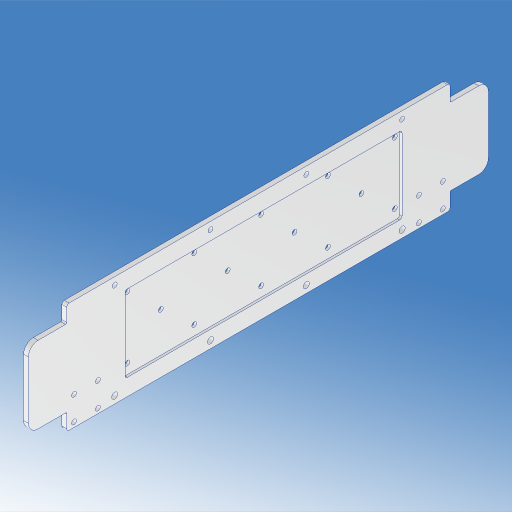
# Autodesk Inventor part: ChassisInterface
Saved by Autodesk Inventor 2024 (Build 280153000, 153)
## iProperties
Created: 2022-11-13
Part Number: ChassisInterface
Material: Aluminum 6061
Document SubType Name: Modeling
Designer: kumpu
Density: 2.7 g/cm^3
Appearance: Aluminum - Flat
Mass: 777.044 g
Surface Area: 1099.09 cm^2
Volume: 287.794 cm^3
Author: kumpu
Autodesk Inventor part; units mm, degrees
ref_plane "YZ Plane" through (0, 0, 0) normal (1, 0, 0) x (0, 1, 0)
ref_plane "XZ Plane" through (0, 0, 0) normal (0, 1, 0) x (-1, 0, 0)
ref_plane "XY Plane" through (0, 0, 0) normal (0, 0, 1) x (1, 0, 0)
sketch "Sketch1" plane through (0, 0, 0) normal (1, 0, 0) x (0, 1, 0)
  line L0 (76.2, 254) -> (-76.2, 254)
  line L1 (-76.2, 254) -> (-76.2, -254)
  line L2 (-76.2, -254) -> (76.2, -254)
  line L3 (76.2, -254) -> (76.2, 254)
  line L4 (76.2, 254) -> (-76.2, -254) construction
  line L5 (-76.2, 254) -> (76.2, -254) construction
  line L6 (50.8, 304.8) -> (-50.8, 304.8)
  line L7 (-50.8, 304.8) -> (-50.8, 254)
  line L8 (-50.8, 254) -> (50.8, 254)
  line L9 (50.8, 254) -> (50.8, 304.8)
  line L10 (50.8, 304.8) -> (-50.8, 254) construction
  line L11 (-50.8, 304.8) -> (50.8, 254) construction
  line L12 (50.8, -254) -> (-50.8, -254)
  line L13 (-50.8, -254) -> (-50.8, -304.8)
  line L14 (-50.8, -304.8) -> (50.8, -304.8)
  line L15 (50.8, -304.8) -> (50.8, -254)
  line L16 (50.8, -254) -> (-50.8, -304.8) construction
  line L17 (-50.8, -254) -> (50.8, -304.8) construction
  line L18 (0, 279.4) -> (0, -279.4) construction
  point P0 (0, 0)
  point P1 (-50.8, -254)
  point P2 (50.8, 254)
  dimension "d0" = 152.4
  dimension "d1" = 508
  dimension "d9" = 50.8
  dimension "d10" = 101.6
  constraints: 38 end point, 7 midpoint, 6 parallel, 3 horizontal, 3 perpendicular, 2 equal length, 1 point on line, 1 vertical
  measures "d0" distance of L2.end L1.end
  measures "d1" distance of L1.end L0.end
  measures "d9" distance of L14.end L12.start
  measures "d10" distance of L13.end L14.end
extrude "Extrusion1" add sketch "Sketch1" along normal mid plane 6.35
sketch "Sketch3" plane through (3.175, 0, 0) normal (1, 0, 0) x (0, 0, -1)
  line L0 (-241.3, 44.45) -> (-201.6125, 44.45)
  line L1 (-201.6125, 44.45) -> (-201.6125, -44.45)
  line L2 (-201.6125, -44.45) -> (-241.3, -44.45)
  line L3 (-241.3, -44.45) -> (-241.3, 44.45)
  line L4 (-179.3875, 44.45) -> (-125.857, 44.45)
  line L5 (-125.857, 44.45) -> (-125.857, -44.45)
  line L6 (-125.857, -44.45) -> (-179.3875, -44.45)
  line L7 (-179.3875, -44.45) -> (-179.3875, 44.45)
  line L8 (-103.632, 44.45) -> (50.8, 44.45)
  line L9 (50.8, 44.45) -> (50.8, -44.45)
  line L10 (50.8, -44.45) -> (-103.632, -44.45)
  line L11 (-103.632, -44.45) -> (-103.632, 44.45)
  line L12 (74.6125, 44.45) -> (179.3875, 44.45)
  line L13 (179.3875, 44.45) -> (179.3875, -44.45)
  line L14 (179.3875, -44.45) -> (74.6125, -44.45)
  line L15 (74.6125, -44.45) -> (74.6125, 44.45)
  line L16 (201.6125, -44.45) -> (241.3, -44.45)
  line L17 (241.3, -44.45) -> (241.3, 44.45)
  line L18 (241.3, 44.45) -> (201.6125, 44.45)
  line L19 (201.6125, 44.45) -> (201.6125, -44.45)
  line L20 (-201.6125, 0) -> (-179.3875, 0) construction
  line L21 (-125.857, 0) -> (-103.632, 0) construction
  line L22 (179.3875, 0) -> (201.6125, 0) construction
  line L23 (-254, -50.8) -> (-254, -76.2) construction
  circle A0 centre (-190.5, 63.5) radius 3.175
  line L24 (-190.5, 63.5) -> (-190.5, 0) construction
  line L25 (-190.5, 0) -> (-190.5, -63.5) construction
  circle A1 centre (-190.5, -63.5) radius 3.9751
  circle A2 centre (-63.5, 63.5) radius 3.175
  circle A3 centre (-63.5, -63.5) radius 3.9751
  circle A4 centre (63.5, 63.5) radius 3.175
  circle A5 centre (63.5, -63.5) radius 3.9751
  circle A6 centre (190.5, 63.5) radius 3.175
  circle A7 centre (190.5, -63.5) radius 3.9751
  line L26 (-125.857, 44.45) -> (-103.632, 44.45)
  line L27 (-103.632, 44.45) -> (-103.632, -44.45)
  line L28 (-103.632, -44.45) -> (-125.857, -44.45)
  line L29 (-125.857, -44.45) -> (-125.857, 44.45)
  line L30 (254, -76.2) -> (254, -50.8) projected
  line L31 (-254, -76.2) -> (254, -76.2) projected
  point P0 (0, 0)
  point P1 (0, 0)
  point P2 (-114.7445, 0)
  dimension "d12" = 22.225
  dimension "d13" = 12.7
  dimension "d14" = 88.9
  dimension "d16" = 6.35
  dimension "d17" = 7.9502
  dimension "d20" = 127
  dimension "d29" = 12.7
  dimension "d30" = 63.5
  dimension "d31" = 12.7
  dimension "d32" = 11.1125
  dimension "d33" = 31.75
  dimension "d34" = 127
  dimension "d35" = 63.5
  dimension "d39" = 154.432
  constraints: 58 end point, 12 parallel, 8 centre point, 8 midpoint, 7 collinear, 7 horizontal, 7 perpendicular, 4 point on line, 2 coincident, 1 vertical, 12 other
  measures "d12" distance of L20.start L20.end
  measures "d13" distance between parallel lines of L23 L3
  measures "d14" distance of L2.end L0.start
  measures "d16" diameter of A0
  measures "d17" diameter of A1
  measures "d20" distance of L24.start A2.centre
  measures "d29" distance from line of L9 A4.centre
  measures "d30" distance between parallel lines of L23 L25
  measures "d31" distance between parallel lines of L30 L17
  measures "d32" distance from line of A4.centre L15
  measures "d33" distance between parallel lines of L31 L2
  measures "d34" distance of L25.end L24.start
  measures "d35" distance from line of L20 L24.start
  measures "d39" distance between parallel lines of L9 L27
extrude "Extrusion3" [suppressed]
fillet "Fillet1" radius 12.7 4 edges at (0, 50.8, 304.8) (0, -50.8, 304.8) (0, 50.8, -304.8) (0, -50.8, -304.8)
fillet "Fillet1" radius 1.5875 8 edges at (0, 50.8, 254) (0, -50.8, 254) (0, -76.2, 254) (0, 76.2, 254) (0, 76.2, -254) (0, 50.8, -254) (0, -50.8, -254) (0, -76.2, -254)
sketch "Sketch4" plane through (-3.175, 0, 0) normal (-1, 0, 0) x (0, 0, 1)
  line L0 (-182.626, 63.5635) -> (-141.351, 63.5635) construction
  line L1 (-254, 74.6125) -> (-254, 52.3875) construction
  line L2 (252.4125, 76.2) -> (-252.4125, 76.2) construction
  point P0 (0, 0)
  dimension "d36" = 71.374
  dimension "d37" = 12.6365
  dimension "d38" = 41.275
  constraints: 2 end point, 1 horizontal
  measures "d36" distance from line of L1 L0.start
  measures "d37" distance between parallel lines of L2 L0
  measures "d38" distance of L0.start L0.end
extrude "Extrusion4" cut sketch "Sketch3" against normal through all contours A0 | A1 | A2 | A3 | A4 | A5 | A6 | A7
sketch "Sketch6" plane through (3.175, 0, 0) normal (1, 0, 0) x (0, 0, -1)
  circle A0 centre (63.5, 63.5) radius 3.175 projected
  circle A1 centre (-63.5, -63.5) radius 3.9751 projected
  circle A2 centre (63.5, -63.5) radius 3.9751 projected
  circle A3 centre (-63.5, 63.5) radius 3.175 projected
  circle A4 centre (190.5, 63.5) radius 3.175 projected
  circle A5 centre (-190.5, -63.5) radius 3.9751 projected
  circle A6 centre (190.5, -63.5) radius 3.9751 projected
  circle A7 centre (-190.5, 63.5) radius 3.175 projected
  arc A8 (252.4125, -76.2) -> (254, -74.6125) centre (252.4125, -74.6125) ccw projected
  line L0 (254, -74.6125) -> (254, -52.3875) projected
  arc A9 (255.5875, -50.8) -> (254, -52.3875) centre (255.5875, -52.3875) ccw projected
  line L1 (255.5875, -50.8) -> (292.1, -50.8) projected
  arc A10 (292.1, -50.8) -> (304.8, -38.1) centre (292.1, -38.1) ccw projected
  line L2 (304.8, -38.1) -> (304.8, 38.1) projected
  arc A11 (304.8, 38.1) -> (292.1, 50.8) centre (292.1, 38.1) ccw projected
  line L3 (292.1, 50.8) -> (255.5875, 50.8) projected
  arc A12 (254, 52.3875) -> (255.5875, 50.8) centre (255.5875, 52.3875) ccw projected
  line L4 (254, 52.3875) -> (254, 74.6125) projected
  arc A13 (254, 74.6125) -> (252.4125, 76.2) centre (252.4125, 74.6125) ccw projected
  line L5 (252.4125, 76.2) -> (-252.4125, 76.2) projected
  arc A14 (-252.4125, 76.2) -> (-254, 74.6125) centre (-252.4125, 74.6125) ccw projected
  line L6 (-254, 74.6125) -> (-254, 52.3875) projected
  arc A15 (-255.5875, 50.8) -> (-254, 52.3875) centre (-255.5875, 52.3875) ccw projected
  line L7 (-255.5875, 50.8) -> (-292.1, 50.8) projected
  arc A16 (-292.1, 50.8) -> (-304.8, 38.1) centre (-292.1, 38.1) ccw projected
  line L8 (-304.8, 38.1) -> (-304.8, -38.1) projected
  arc A17 (-304.8, -38.1) -> (-292.1, -50.8) centre (-292.1, -38.1) ccw projected
  line L9 (-292.1, -50.8) -> (-255.5875, -50.8) projected
  arc A18 (-254, -52.3875) -> (-255.5875, -50.8) centre (-255.5875, -52.3875) ccw projected
  line L10 (-254, -52.3875) -> (-254, -74.6125) projected
  arc A19 (-254, -74.6125) -> (-252.4125, -76.2) centre (-252.4125, -74.6125) ccw projected
  line L11 (-252.4125, -76.2) -> (252.4125, -76.2) projected
  line L12 (-292.1, 47.625) -> (-255.5875, 47.625)
  arc A20 (-255.5875, 47.625) -> (-250.825, 52.3875) centre (-255.5875, 52.3875) ccw
  line L13 (-250.825, 52.3875) -> (-250.825, 73.025)
  line L14 (-250.825, 73.025) -> (250.825, 73.025)
  line L15 (250.825, 73.025) -> (250.825, 52.3875)
  arc A21 (250.825, 52.3875) -> (255.5875, 47.625) centre (255.5875, 52.3875) ccw
  line L16 (255.5875, 47.625) -> (292.1, 47.625)
  arc A22 (301.625, 38.1) -> (292.1, 47.625) centre (292.1, 38.1) ccw
  line L17 (301.625, 38.1) -> (301.625, -38.1)
  arc A23 (292.1, -47.625) -> (301.625, -38.1) centre (292.1, -38.1) ccw
  line L18 (292.1, -47.625) -> (255.5875, -47.625)
  arc A24 (255.5875, -47.625) -> (250.825, -52.3875) centre (255.5875, -52.3875) ccw
  line L19 (250.825, -52.3875) -> (250.825, -73.025)
  line L20 (250.825, -73.025) -> (-250.825, -73.025)
  line L21 (-250.825, -73.025) -> (-250.825, -52.3875)
  arc A25 (-250.825, -52.3875) -> (-255.5875, -47.625) centre (-255.5875, -52.3875) ccw
  line L22 (-255.5875, -47.625) -> (-292.1, -47.625)
  arc A26 (-301.625, -38.1) -> (-292.1, -47.625) centre (-292.1, -38.1) ccw
  line L23 (-301.625, -38.1) -> (-301.625, 38.1)
  arc A27 (-292.1, 47.625) -> (-301.625, 38.1) centre (-292.1, 38.1) ccw
  line L24 (-295.0658, 0) -> (-301.625, 0) construction
  line L25 (-176.784, 50.8) -> (190.3494, 50.8)
  line L26 (190.3494, 50.8) -> (190.3494, -50.8)
  line L27 (190.3494, -50.8) -> (-176.784, -50.8)
  line L28 (-176.784, -50.8) -> (-176.784, 50.8)
  line L29 (-254, -50.8) -> (254, -50.8) construction
  line L30 (254, -50.8) -> (254, -76.2) construction
  line L31 (254, -76.2) -> (-254, -76.2) construction
  line L32 (-254, -76.2) -> (-254, -50.8) construction
  line L33 (-254, 76.2) -> (254, 76.2) construction
  line L34 (254, 76.2) -> (254, 50.8) construction
  line L35 (254, 50.8) -> (-254, 50.8) construction
  line L36 (-254, 50.8) -> (-254, 76.2) construction
  circle A28 centre (-170.434, 44.45) radius 3.302
  circle A29 centre (183.9994, 44.45) radius 3.175
  circle A30 centre (-81.8256, 44.45) radius 3.175
  circle A31 centre (6.7827, 44.45) radius 3.175
  circle A32 centre (95.3911, 44.45) radius 3.175
  line L37 (-330.2, 73.025) -> (-330.2, -50.8) construction
  circle A33 centre (-37.5215, 1.7998) radius 3.175
  circle A34 centre (51.0869, 1.7998) radius 3.175
  line L38 (639.9011, -38.0592) -> (645.7898, -37.8143) construction
  circle A35 centre (228.6, -50.8) radius 12.7 construction
  circle A36 centre (-228.6, -50.8) radius 12.7 construction
  circle A37 centre (-228.6, -50.8) radius 15.875 construction
  line L39 (-244.475, -34.925) -> (-212.725, -34.925) construction
  line L40 (-212.725, -34.925) -> (-212.725, -66.675) construction
  line L41 (-212.725, -66.675) -> (-244.475, -66.675) construction
  line L42 (-244.475, -66.675) -> (-244.475, -34.925) construction
  circle A38 centre (228.6, -50.8) radius 15.875 construction
  line L43 (212.725, -34.925) -> (244.475, -34.925) construction
  line L44 (244.475, -34.925) -> (244.475, -66.675) construction
  line L45 (244.475, -66.675) -> (212.725, -66.675) construction
  line L46 (212.725, -66.675) -> (212.725, -34.925) construction
  circle A39 centre (-244.475, -34.925) radius 3.175
  circle A40 centre (-244.475, -66.675) radius 3.175
  circle A41 centre (-212.725, -66.675) radius 3.175
  circle A42 centre (-212.725, -34.925) radius 3.175
  circle A43 centre (212.725, -34.925) radius 3.175
  circle A44 centre (244.475, -34.925) radius 3.175
  circle A45 centre (212.725, -66.675) radius 3.175
  circle A46 centre (244.475, -66.675) radius 3.175
  line L47 (643.6065, -35.788) -> (639.9011, -38.0592) construction
  line L48 (6.7827, 50.8) -> (6.7827, -50.8) construction
  circle A47 centre (-126.1298, 1.7998) radius 3.175
  circle A48 centre (139.6953, 1.7998) radius 3.175
  circle A49 centre (-37.5215, 1.7998) radius 3.175
  circle A50 centre (51.0869, 1.7998) radius 3.175
  circle A51 centre (-126.1298, 1.7998) radius 3.175
  circle A52 centre (139.6953, 1.7998) radius 3.175
  circle A53 centre (-170.434, -37.6754) radius 3.175
  circle A54 centre (-81.8256, -37.6754) radius 3.175
  circle A55 centre (6.7827, -37.6754) radius 3.175
  circle A56 centre (95.3911, -37.6754) radius 3.175
  circle A57 centre (183.9994, -37.6754) radius 3.175
  dimension "d42" = 3.175
  dimension "d57" = 101.6
  dimension "d58" = 25.4
  dimension "d59" = 25.4
  dimension "d60" = 367.1334
  dimension "d61" = 6.35
  dimension "d62" = 6.35
  dimension "d63" = 6.35
  dimension "d64" = 6.35
  dimension "d65" = 6.604
  dimension "d66" = 6.35
  dimension "d69" = 6.35
  dimension "d70" = 6.35
  dimension "d71" = 6.35
  dimension "d73" = 25.4
  dimension "d82" = 6.35
  dimension "d84" = 6.35
  dimension "d119" = 25.4
  dimension "d120" = 25.4
  dimension "d121" = 76.2
  dimension "d124" = 25.4
  dimension "d125" = 76.2
  dimension "d126" = 25.4
  dimension "d127" = 3.175
  dimension "d128" = 3.175
  dimension "d129" = 6.35
  dimension "d130" = 6.35
  dimension "d131" = 6.35
  dimension "d132" = 6.35
  dimension "d133" = 6.35
  dimension "d134" = 6.35
  dimension "d135" = 6.35
  dimension "d136" = 6.35
  dimension "d139" = 177.2167
  dimension "d140" = 88.6084
  dimension "d141" = 88.6084
  dimension "d142" = 6.35
  dimension "d143" = 6.35
  dimension "d144" = 44.3042
  dimension "d145" = 44.3042
  dimension "d146" = 44.3042
  dimension "d147" = 44.3042
  dimension "d148" = 38.2506
  dimension "d149" = 6.35
  dimension "d151" = 6.35
  dimension "d152" = 6.35
  dimension "d153" = 6.35
  dimension "d154" = 6.35
  dimension "d155" = 42.6502
  dimension "d156" = 82.1254
  constraints: 74 end point, 38 centre point, 16 point on circle, 10 horizontal alignment, 10 parallel, 8 coincident, 8 tangent, 7 collinear, 6 horizontal, 5 perpendicular, 4 vertical alignment, 3 midpoint, 2 point on line, 1 vertical, 19 other
  measures "d42" distance between parallel lines of L7 L12
  measures "d57" distance of L25.end L26.end
  measures "d58" distance of L29.end L30.end
  measures "d59" distance of L35.end L33.start
  measures "d60" distance between parallel lines of L26 L28
  measures "d61" distance from line of L28 A28.centre
  measures "d62" distance from line of L35 A28.centre
  measures "d63" distance from line of L25 A29.centre
  measures "d64" distance from line of L26 A29.centre
  measures "d65" diameter of A28
  measures "d66" diameter of A29
  measures "d69" diameter of A30
  measures "d70" diameter of A31
  measures "d71" diameter of A32
  measures "d73" distance between parallel lines of L8 L37
  measures "d82" diameter of A33
  measures "d84" diameter of A34
  measures "d119" diameter of A35
  measures "d120" distance from line of L11 A35.centre
  measures "d121" distance from line of A35.centre L2
  measures "d124" diameter of A36
  measures "d125" distance from line of A36.centre L8
  measures "d126" distance from line of L11 A36.centre
  measures "d127" radial gap between concentric circles of A36 A37
  measures "d128" radial gap between concentric circles of A35 A38
  measures "d129" diameter of A39
  measures "d130" diameter of A40
  measures "d131" diameter of A41
  measures "d132" diameter of A42
  measures "d133" diameter of A43
  measures "d134" diameter of A44
  measures "d135" diameter of A45
  measures "d136" diameter of A46
  measures "d139" distance of A31.centre A28.centre
  measures "d140" distance of A30.centre A28.centre
  measures "d141" distance of A32.centre A31.centre
  measures "d142" diameter of A47
  measures "d143" diameter of A48
  measures "d144" horizontal distance of A47.centre A28.centre
  measures "d145" horizontal distance of A33.centre A30.centre
  measures "d146" horizontal distance of A34.centre A31.centre
  measures "d147" horizontal distance of A48.centre A32.centre
  measures "d148" distance from line of A35.centre L26
  measures "d149" diameter of A53
  measures "d151" diameter of A54
  measures "d152" diameter of A55
  measures "d153" diameter of A56
  measures "d154" diameter of A57
  measures "d155" vertical distance of A47.centre A28.centre
  measures "d156" distance of A53.centre A28.centre
extrude "Extrusion5" cut sketch "Sketch6" against normal blind 25.4 contours A28 | A29 | A30 | A31 | A32 | A33 | A34 | A47 | A48 | A53 | A54 | A55 | A56 | A57
extrude "Extrusion6" cut sketch "Sketch6" against normal blind 3.175 contours L25 L26 L27 L28 | A28 | A29 | A30 | A31 | A32 | A33 | A34 | A47 | A48 | A53 | A54 | A55 | A56 | A57
sketch "Sketch7" plane through (3.175, 0, 0) normal (1, 0, 0) x (0, 0, -1)
  line L0 (190.3494, 50.8) -> (190.3494, -50.8) projected
  line L1 (190.3494, -50.8) -> (-176.784, -50.8) projected
  line L2 (-176.784, -50.8) -> (-176.784, 50.8) projected
  line L3 (-176.784, 50.8) -> (190.3494, 50.8) projected
  circle A0 centre (63.5, 63.5) radius 3.175 projected
  circle A1 centre (-63.5, -63.5) radius 3.9751 projected
  circle A2 centre (63.5, -63.5) radius 3.9751 projected
  circle A3 centre (-63.5, 63.5) radius 3.175 projected
  circle A4 centre (190.5, 63.5) radius 3.175 projected
  circle A5 centre (-190.5, -63.5) radius 3.9751 projected
  circle A6 centre (190.5, -63.5) radius 3.9751 projected
  circle A7 centre (-190.5, 63.5) radius 3.175 projected
  arc A8 (252.4125, -76.2) -> (254, -74.6125) centre (252.4125, -74.6125) ccw projected
  line L4 (254, -74.6125) -> (254, -52.3875) projected
  arc A9 (255.5875, -50.8) -> (254, -52.3875) centre (255.5875, -52.3875) ccw projected
  line L5 (255.5875, -50.8) -> (292.1, -50.8) projected
  arc A10 (292.1, -50.8) -> (304.8, -38.1) centre (292.1, -38.1) ccw projected
  line L6 (304.8, -38.1) -> (304.8, 38.1) projected
  arc A11 (304.8, 38.1) -> (292.1, 50.8) centre (292.1, 38.1) ccw projected
  line L7 (292.1, 50.8) -> (255.5875, 50.8) projected
  arc A12 (254, 52.3875) -> (255.5875, 50.8) centre (255.5875, 52.3875) ccw projected
  line L8 (254, 52.3875) -> (254, 74.6125) projected
  arc A13 (254, 74.6125) -> (252.4125, 76.2) centre (252.4125, 74.6125) ccw projected
  line L9 (252.4125, 76.2) -> (-252.4125, 76.2) projected
  arc A14 (-252.4125, 76.2) -> (-254, 74.6125) centre (-252.4125, 74.6125) ccw projected
  line L10 (-254, 74.6125) -> (-254, 52.3875) projected
  arc A15 (-255.5875, 50.8) -> (-254, 52.3875) centre (-255.5875, 52.3875) ccw projected
  line L11 (-255.5875, 50.8) -> (-292.1, 50.8) projected
  arc A16 (-292.1, 50.8) -> (-304.8, 38.1) centre (-292.1, 38.1) ccw projected
  line L12 (-304.8, 38.1) -> (-304.8, -38.1) projected
  arc A17 (-304.8, -38.1) -> (-292.1, -50.8) centre (-292.1, -38.1) ccw projected
  line L13 (-292.1, -50.8) -> (-255.5875, -50.8) projected
  arc A18 (-254, -52.3875) -> (-255.5875, -50.8) centre (-255.5875, -52.3875) ccw projected
  line L14 (-254, -52.3875) -> (-254, -74.6125) projected
  arc A19 (-254, -74.6125) -> (-252.4125, -76.2) centre (-252.4125, -74.6125) ccw projected
  line L15 (-252.4125, -76.2) -> (252.4125, -76.2) projected
  line L16 (-250.825, 52.3875) -> (-250.825, 73.025)
  line L17 (-250.825, 73.025) -> (250.825, 73.025)
  line L18 (250.825, 73.025) -> (250.825, 52.3875)
  arc A20 (250.825, 52.3875) -> (255.5875, 47.625) centre (255.5875, 52.3875) ccw
  line L19 (255.5875, 47.625) -> (292.1, 47.625)
  arc A21 (301.625, 38.1) -> (292.1, 47.625) centre (292.1, 38.1) ccw
  line L20 (301.625, 38.1) -> (301.625, -38.1)
  arc A22 (292.1, -47.625) -> (301.625, -38.1) centre (292.1, -38.1) ccw
  line L21 (292.1, -47.625) -> (255.5875, -47.625)
  arc A23 (255.5875, -47.625) -> (250.825, -52.3875) centre (255.5875, -52.3875) ccw
  line L22 (250.825, -52.3875) -> (250.825, -73.025)
  line L23 (250.825, -73.025) -> (-250.825, -73.025)
  line L24 (-250.825, -73.025) -> (-250.825, -52.3875)
  arc A24 (-250.825, -52.3875) -> (-255.5875, -47.625) centre (-255.5875, -52.3875) ccw
  line L25 (-255.5875, -47.625) -> (-292.1, -47.625)
  arc A25 (-301.625, -38.1) -> (-292.1, -47.625) centre (-292.1, -38.1) ccw
  line L26 (-301.625, -38.1) -> (-301.625, 38.1)
  arc A26 (-292.1, 47.625) -> (-301.625, 38.1) centre (-292.1, 38.1) ccw
  line L27 (-292.1, 47.625) -> (-255.5875, 47.625)
  arc A27 (-255.5875, 47.625) -> (-250.825, 52.3875) centre (-255.5875, 52.3875) ccw
  line L28 (196.6994, 57.15) -> (196.6994, -57.15)
  line L29 (196.6994, -57.15) -> (-183.134, -57.15)
  line L30 (-183.134, -57.15) -> (-183.134, 57.15)
  line L31 (-183.134, 57.15) -> (196.6994, 57.15)
  circle A28 centre (-190.5, 63.5) radius 6.35
  circle A29 centre (-63.5, 63.5) radius 6.35
  circle A30 centre (63.5, 63.5) radius 6.35
  circle A31 centre (190.5, 63.5) radius 6.35
  circle A32 centre (-190.5, -63.5) radius 6.35
  circle A33 centre (-63.5, -63.5) radius 6.35
  circle A34 centre (63.5, -63.5) radius 6.35
  circle A35 centre (190.5, -63.5) radius 6.35
  point P0 (0, 0)
  dimension "d116" = 3.175
  dimension "d117" = 6.35
  dimension "d118" = 3.175
  constraints: 32 end point, 16 centre point, 16 point on circle, 7 equal radius, 22 other
  measures "d116" distance between parallel lines of L10 L16
  measures "d117" distance between parallel lines of L3 L31
  measures "d118" radial gap between concentric circles of A7 A28
fillet "Fillet2" radius 3.175 4 edges at (1.5875, 50.8, 176.784) (1.5875, -50.8, 176.784) (1.5875, -50.8, -190.3494) (1.5875, 50.8, -190.3494)
extrude "Extrusion7" cut sketch "Sketch6" against normal blind 25.4 contours A39 | A40 | A41 | A42 | A43 | A44 | A45 | A46
sketch "Sketch9" plane through (3.175, 0, 0) normal (1, 0, 0) x (0, 0, -1)
  line L0 (-254, 74.6125) -> (-254, 52.3875) projected
  line L1 (-254, 73.025) -> (254, 73.025)
  line L2 (254, 52.3875) -> (254, 74.6125) projected
  line L3 (252.4125, 76.2) -> (-252.4125, 76.2) projected
  line L4 (-254, -52.3875) -> (-254, -74.6125) projected
  line L5 (-254, -73.025) -> (254, -73.025)
  line L6 (254, -52.3875) -> (254, -74.6125) projected
  line L7 (-252.4125, -76.2) -> (252.4125, -76.2) projected
  arc A0 (-252.4125, 76.2) -> (-254, 74.6125) centre (-252.4125, 74.6125) ccw projected
  arc A1 (254, 74.6125) -> (252.4125, 76.2) centre (252.4125, 74.6125) ccw projected
  arc A2 (252.4125, -76.2) -> (254, -74.6125) centre (252.4125, -74.6125) ccw projected
  arc A3 (-254, -74.6125) -> (-252.4125, -76.2) centre (-252.4125, -74.6125) ccw projected
  point P0 (0, 0)
  dimension "d157" = 3.175
  dimension "d158" = 3.175
  constraints: 4 end point, 4 point on line, 2 horizontal
  measures "d157" distance between parallel lines of L3 L1
  measures "d158" distance between parallel lines of L7 L5
extrude "Extrusion8" cut sketch "Sketch9" against normal blind 25.4
fillet "Fillet3" radius 3.175 4 edges at (0, 73.025, 254) (0, 73.025, -254) (0, -73.025, -254) (0, -73.025, 254)
body "Solid1"
